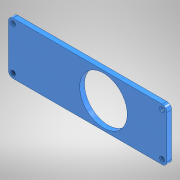
# Autodesk Inventor part: 덮개
Saved by Autodesk Inventor 2022 (Build 260153000, 153)
## iProperties
Created: 2024-07-11
Part Number: 덮개
Material: 일반
Document SubType Name: Modeling
Designer: seama
Density: 1 g/cm^3
Appearance: 시안색
Author: seama
Autodesk Inventor part; units mm, degrees
ref_plane "우측면도" through (0, 0, 0) normal (1, 0, 0) x (0, 1, 0)
ref_plane "평면도" through (0, 0, 0) normal (0, 1, 0) x (-1, 0, 0)
ref_plane "정면도" through (0, 0, 0) normal (0, 0, 1) x (1, 0, 0)
sketch "스케치1" plane through (0, 0, 0) normal (0, 0, 1) x (1, 0, 0)
  line L0 (0, 0) -> (100, 0)
  line L1 (100, 0) -> (100, 33)
  line L2 (100, 33) -> (0, 33)
  line L3 (0, 33) -> (0, 0)
  dimension "d0" = 100
  dimension "d1" = 33
  constraints: 8 end point, 2 parallel, 1 horizontal, 1 perpendicular
  measures "d0" distance of L0.start L0.end
  measures "d1" distance of L0.end L1.end
extrude "돌출1" add sketch "스케치1" along normal blind 3
fillet "모깎기1" radius 3 4 edges at (0, 33, 1.5) (0, 0, 1.5) (100, 0, 1.5) (100, 33, 1.5)
sketch "스케치2" plane through (0, 0, 3) normal (0, 0, 1) x (1, 0, 0)
  circle A0 centre (3, 30) radius 1.5
  circle A1 centre (3, 30) radius 3
  line L0 (100, 33) -> (0, 33) projected
  line L1 (0, 33) -> (0, 0) projected
  circle A2 centre (97, 30) radius 1.5
  circle A3 centre (97, 30) radius 3
  circle A4 centre (3, 3) radius 1.5
  circle A5 centre (3, 3) radius 3
  circle A6 centre (97, 3) radius 1.5
  circle A7 centre (97, 3) radius 3
  dimension "d4" = 3
  dimension "d5" = 6
  dimension "d8" = 94
  dimension "d11" = 27
  constraints: 8 centre point, 4 coincident, 2 tangent, 1 horizontal, 1 vertical, 12 other
  measures "d4" diameter of A0
  measures "d5" diameter of A1
  measures "d8" distance of A0.centre A2.centre
  measures "d11" distance of A0.centre A4.centre
extrude "돌출2" cut sketch "스케치2" against normal blind 4 contours A0 | A2 | A4 | A6
sketch "스케치3" plane through (0, 0, 3) normal (0, 0, 1) x (1, 0, 0)
  line L0 (45, 31.5) -> (75, 31.5) construction
  line L1 (75, 31.5) -> (75, 1.5) construction
  line L2 (75, 1.5) -> (45, 1.5) construction
  line L3 (45, 1.5) -> (45, 31.5) construction
  line L4 (100, 3) -> (100, 30) projected
  line L5 (3, 0) -> (97, 0) projected
  line L6 (97, 33) -> (3, 33) projected
  circle A0 centre (60, 16.5) radius 15
  point P0 (0, 0)
  dimension "d28" = 25
  dimension "d29" = 1.5
  dimension "d30" = 1.5
  dimension "d33" = 30
  constraints: 8 end point, 4 tangent, 2 parallel, 1 centre point, 1 horizontal, 1 perpendicular
  measures "d28" distance between parallel lines of L4 L1
  measures "d29" distance between parallel lines of L5 L2
  measures "d30" distance between parallel lines of L6 L0
  measures "d33" diameter of A0
extrude "돌출3" cut sketch "스케치3" against normal blind 4
equation "\"d8\" = d0 - d5"
equation "\"d11\" = d1 - d5"
equation "\"d30\" = d29"
